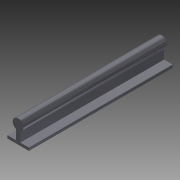
# Autodesk Inventor part: z rail
Saved by Autodesk Inventor 2012 (Build 160160000, 160)
## iProperties
Created: 2013-05-09
Part Number: z rail
Material: Default
Document SubType Name: Modeling
Designer: Fabian
Density: 1 g/cm^3
Author: Fabian
Autodesk Inventor part; units mm, degrees
ref_plane "YZ Plane" through (0, 0, 0) normal (1, 0, 0) x (0, 1, 0)
ref_plane "XZ Plane" through (0, 0, 0) normal (0, 1, 0) x (-1, 0, 0)
ref_plane "XY Plane" through (0, 0, 0) normal (0, 0, 1) x (1, 0, 0)
sketch "Sketch1" plane through (0, 0, 0) normal (0, 0, 1) x (1, 0, 0)
  circle A0 centre (-6.6643, 9.7203) radius 7.5
  line L0 (-9.6643, 9.7203) -> (-3.6643, 9.7203)
  line L1 (-3.6643, 9.7203) -> (-3.6643, -10.5455)
  line L2 (-3.6643, -10.5455) -> (-9.6643, -10.5455)
  line L3 (-9.6643, -10.5455) -> (-9.6643, 9.7203)
  line L4 (-21.6643, -10.5455) -> (8.3357, -10.5455)
  line L5 (8.3357, -10.5455) -> (8.3357, -14.5455)
  line L6 (8.3357, -14.5455) -> (-21.6643, -14.5455)
  line L7 (-21.6643, -14.5455) -> (-21.6643, -10.5455)
  point P0 (0, 0)
  point P1 (0, 0)
  dimension "d0" = 15
  dimension "d1" = 6
  dimension "d2" = 4
  dimension "d3" = 30
  dimension "d4" = 12
  dimension "d5" = 3
  dimension "d6" = 3
  dimension "d7" = 12
  dimension "d8" = 0
  constraints: 16 end point, 4 parallel, 2 horizontal, 2 perpendicular, 1 centre point
  measures "d0" diameter of A0
  measures "d1" distance of L0.start L0.end
  measures "d2" distance of L4.end L5.end
  measures "d3" distance of L5.end L6.end
  measures "d4" distance between parallel lines of L7 L3
  measures "d5" distance from line of A0.centre L3
  measures "d6" distance from line of A0.centre L1
  measures "d7" distance between parallel lines of L5 L1
  measures "d8" distance between parallel lines of L4 L2
extrude "Extrusion1" add sketch "Sketch1" along normal blind 200
equation "\"d4\" = d7"
body "Solid1"
